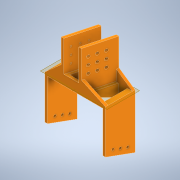
# Autodesk Inventor part: bracketForGarageV02
Saved by Autodesk Inventor 2022.1 (Build 261234020, 234B)
## iProperties
Created: 2021-10-20
Part Number: bracketForGarageV02
Material: PC/ABS Plastic
Document SubType Name: Modeling
Designer: robst
Density: 0.357273 g/cm^3
Appearance: Orange
Author: robst
Autodesk Inventor part; units mm, degrees
note: some values were not read from the file. Chosen so that the rebuilt part matches the saved one: direction of "HoleForLeftSideOf2x4"; direction of "HolesForRightSideOf2x4".
ref_plane "YZ Plane" through (0, 0, 0) normal (1, 0, 0) x (0, 1, 0)
ref_plane "XY Plane" through (0, 0, 0) normal (0, 0, 1) x (1, 0, 0)
sketch "Sketch8" plane through (0, 0, 0) normal (0, 1, 0) x (-1, 0, 0)
  line L0 (82, 40) -> (-82, 40)
  line L1 (-82, 40) -> (-82, -40)
  line L2 (-82, -40) -> (82, -40)
  line L3 (82, -40) -> (82, 40)
  line L4 (82, 40) -> (-82, -40) construction
  line L5 (-82, 40) -> (82, -40) construction
  point P0 (0, 0)
  dimension "d28" = 80
  dimension "d29" = 164
  constraints: 12 end point, 2 midpoint, 2 parallel, 1 horizontal, 1 perpendicular
  measures "d28" distance of L2.end L0.start
  measures "d29" distance between parallel lines of L1 L3
extrude "Extrusion8" add sketch "Sketch8" against normal blind 7
sketch "Sketch9" plane through (0, -7, 0) normal (0, -1, 0) x (1, 0, 0)
  line L0 (82, 40) -> (-82, 40) projected
  line L1 (-82, -40) -> (82, -40) projected
  line L2 (-82, 40) -> (-75, 40)
  line L3 (-75, 40) -> (-75, -40)
  line L4 (-75, -40) -> (-82, -40)
  line L5 (-82, -40) -> (-82, 40)
  line L6 (82, -40) -> (82, 40) projected
  line L7 (82, -40) -> (75, -40)
  line L8 (75, -40) -> (75, 40)
  line L9 (75, 40) -> (82, 40)
  line L10 (82, 40) -> (82, -40)
  point P0 (0, 0)
  point P1 (75, 40)
  point P2 (75, -40)
  point P3 (-82, -40)
  dimension "d32" = 7
  dimension "d33" = 7
  constraints: 16 end point, 4 parallel, 2 horizontal, 2 perpendicular, 2 point on line
  measures "d32" distance between parallel lines of L3 L5
  measures "d33" distance between parallel lines of L6 L8
extrude "armsForCameraCase" add sketch "Sketch9" along normal blind 140 contours L6 L1 L8 L0 | L3 L1 L5 L0
sketch "Sketch10" plane through (-75, -7, 40) normal (1, 0, 0) x (0, 0, -1)
  line L0 (0, 0) -> (80, 0)
  line L1 (80, 0) -> (80, -140)
  line L2 (80, -140) -> (0, -140)
  line L3 (0, 0) -> (0, -140)
  line L4 (0, 0) -> (80, -29.117619)
  line L5 (80, -29.117619) -> (80, 0)
  line L6 (80, 0) -> (0, 0)
  point P0 (40, 7)
  point P1 (40, -14.558809)
  dimension "d48" = 20
  constraints: 6 end point, 2 collinear, 1 midpoint, 1 point on line
  measures "d48" angle of L4 L0
extrude "Extrusion10" add sketch "Sketch10" along normal up to surface (150 mm away) contours L0 L1 L4
sketch "Sketch11" plane through (0, 0, 0) normal (0, 1, 0) x (1, 0, 0)
  line L0 (82, 40) -> (-82, 40)
  line L1 (-82, -40) -> (82, -40)
  line L2 (-82, 40) -> (-82, -40)
  line L3 (82, -40) -> (82, 40)
  line L4 (-31.037968, -40) -> (-9.602032, 40)
  line L5 (-9.602032, 40) -> (-16.848966, 40)
  line L6 (-75, 40) -> (75, 40)
  line L7 (-16.848966, 40) -> (-38.284901, -40)
  line L8 (-38.284901, -40) -> (-31.037968, -40)
  line L9 (-31.037968, -40) -> (-31.037968, 40) construction
  line L10 (0, -40) -> (0, 40) construction
  line L11 (9.602032, -40) -> (31.037968, 40)
  line L12 (31.037968, 40) -> (38.284901, 40)
  line L13 (38.284901, 40) -> (16.848966, -40)
  line L14 (16.848966, -40) -> (9.602032, -40)
  point P0 (0, 0)
  point P1 (0, -40)
  point P2 (0, -40)
  point P3 (-20.32, 0)
  point P4 (0, 0)
  point P5 (20.32, 0)
  point P6 (38.284901, 40)
  point P7 (31.037968, 40)
  point P8 (-16.848966, 40)
  dimension "d39" = -15
  dimension "d40" = 7
  dimension "d42" = 7
  dimension "d44" = 20.32
  dimension "d45" = 20.32
  constraints: 20 end point, 5 point on line, 4 midpoint, 3 parallel, 2 horizontal, 1 perpendicular, 8 other
  measures "d39" angle of L4 L9
  measures "d40" distance between parallel lines of L7 L4
  measures "d42" distance between parallel lines of L13 L11
  measures "d44" distance of point (-20.32, 0) point (0, 0)
  measures "d45" distance of point (20.32, 0) point (0, 0)
extrude "Extrusion11" add sketch "Sketch11" along normal blind 104.1375 contours L13 L1 L11 L0 | L4 L1 L7 L0
sketch "Sketch12" plane through (0, 0, 0) normal (0, 1, 0) x (1, 0, 0)
  line L0 (31.037968, 40) -> (-9.602032, 40)
  line L1 (31.037968, 40) -> (9.602032, -40)
  line L2 (-31.037968, -40) -> (9.602032, -40)
  line L3 (-31.037968, -40) -> (-9.602032, 40)
  line L4 (-9.602032, 40) -> (31.037968, 40)
  line L5 (31.037968, 40) -> (9.602032, -40)
  line L6 (9.602032, -40) -> (-31.037968, -40)
  line L7 (-9.602032, 40) -> (-31.037968, -40)
  line L8 (-31.037968, -40) -> (-9.602032, 40)
  point P0 (0, 0)
  constraints: 8 end point, 3 equal length
extrude "Extrusion12" add sketch "Sketch12" along normal blind 20
sketch "Sketch13" plane through (-82, 0, -40) normal (-1, 0, 0) x (0, 0, 1)
  line L0 (0, -36.117619) -> (80, -7)
  line L1 (80, 0) -> (80, -147)
  line L2 (80, -147) -> (0, -147)
  line L3 (0, 0) -> (0, -147)
  line L4 (80, -147) -> (0, -147) construction
  line L5 (40, -147) -> (40, -21.558809) construction
  line L6 (80, -7) -> (0, -36.117619) construction
  line L7 (0, -131.893618) -> (80, -102.776) construction
  line L8 (80, -7) -> (80, -147) construction
  point P0 (40, 0)
  point P1 (40, -117.334809)
  point P2 (20, -124.614214)
  point P3 (60, -110.055404)
  dimension "centerForTwoHoles" = 21.28356
  dimension "d51" = 90
  dimension "diagonalLine" = 85.13422
  dimension "d62" = 21.28356
  dimension "d63" = 21.28356
  constraints: 4 end point, 4 point on line, 3 midpoint, 1 parallel
  measures "d51" distance between parallel lines of L7 L0
  measures "diagonalLine" distance of L7.start L7.end
  measures "d62" distance of point (20, -124.614) L7.start
  measures "d63" distance of point (60, -110.055) L7.end
hole "Hole1" at (-82, -117.334809, 0) at (-82, -124.614214, -20) at (-82, -110.055404, 20) direction (1, 0, 0) diameter 6.7564 end through all clearance for "Hex Machine Screw" size "1/4" standard "Ansi Unified Screw Threads"
sketch "Sketch14" plane through (-82, 0, -40) normal (-1, 0, 0) x (0, 0, 1)
  line L0 (80, 0) -> (80, -147)
  line L1 (80, -147) -> (0, -147)
  line L2 (0, 0) -> (0, -147)
  line L3 (0, -36.117619) -> (80, -7)
  line L4 (0, -36.117619) -> (0, -147)
  line L5 (0, -147) -> (80, -117.882381)
  line L6 (0, -147) -> (80, -147)
  line L7 (0, -147) -> (80, -147)
  line L8 (80, -147) -> (80, -117.882381)
  point P0 (40, 0)
  constraints: 6 end point, 2 collinear, 1 parallel, 1 point on line
extrude "Extrusion13" cut sketch "Sketch14" against normal through all contours L0 L1 L5
sketch "Sketch15" plane through (-38.284901, 0, 40) normal (-0.9659258, 0, -0.258819) x (-0.258819, 0, 0.9659258)
  line L0 (-82.822094, 104.1375) -> (0, 104.1375)
  line L1 (0, 0) -> (0, 104.1375)
  line L2 (-82.822094, 0) -> (-82.822094, 104.1375)
  line L3 (-1.875644, 20) -> (-84.697739, 20)
  line L4 (-82.822094, 40) -> (0, 40) construction
  line L5 (-57.822094, 40) -> (-57.822094, 104.1375) construction
  point P0 (-48.545895, 0)
  point P1 (-82.822094, 52.06875)
  point P2 (-37.822094, 40)
  point P3 (-17.822094, 40)
  point P4 (-57.822094, 60)
  point P5 (-37.822094, 60)
  point P6 (-17.822094, 60)
  point P7 (-57.822094, 80)
  point P8 (-37.822094, 80)
  point P9 (-17.822094, 80)
  dimension "d64" = 25
  dimension "d74" = 20
  dimension "d77" = 20
  dimension "d90" = 20
  constraints: 4 end point, 4 point on line, 2 perpendicular, 1 coincident, 1 horizontal, 1 midpoint, 1 vertical, 8 other
  measures "d64" distance from line of point (-82.822, 52.069) L5
  measures "d74" distance of point (-57.822, 40) point (-37.822, 40)
  measures "d77" distance of point (-57.822, 40) point (-57.822, 60)
  measures "d90" distance between parallel lines of L4 L3
hole "HoleForLeftSideOf2x4" at (-23.319442, 40, -15.851854) at (-28.495823, 40, 3.466662) at (-33.672203, 40, 22.785179) at (-28.495823, 60, 3.466662) at (-23.319442, 60, -15.851854) at (-33.672203, 60, 22.785179) at (-33.672203, 80, 22.785179) at (-28.495823, 80, 3.466662) at (-23.319442, 80, -15.851854) direction (0.9659258, 0, 0.258819) diameter 4.496 depth 7 countersink diameter 8.433 countersink angle 82 clearance for "Flat Head Machine Screw (82)" size "#8" standard "Ansi Unified Screw Threads"
sketch "Sketch16" plane through (38.284901, 0, -40) normal (0.9659258, 0, 0.258819) x (0.258819, 0, -0.9659258)
  line L0 (-82.822094, 104.1375) -> (0, 104.1375)
  line L1 (0, 0) -> (0, 104.1375)
  line L2 (-82.822094, 0) -> (-82.822094, 104.1375)
  line L3 (-82.822094, 0) -> (-65.959766, 0)
  line L4 (-1.875644, 20) -> (-84.697739, 20)
  line L5 (-82.822094, 40) -> (0, 40) construction
  line L6 (-67.822094, 40) -> (-67.822094, 104.1375) construction
  point P0 (-48.545895, 0)
  point P1 (-47.822094, 40)
  point P2 (-27.822094, 40)
  point P3 (-67.822094, 60)
  point P4 (-47.822094, 60)
  point P5 (-27.822094, 60)
  point P6 (-67.822094, 80)
  point P7 (-47.822094, 80)
  point P8 (-27.822094, 80)
  dimension "d80" = 20
  dimension "d81" = 15
  dimension "d84" = 20
  dimension "d87" = 20
  constraints: 4 end point, 4 point on line, 2 perpendicular, 1 coincident, 1 horizontal, 1 vertical, 8 other
  measures "d80" distance between parallel lines of L5 L4
  measures "d81" distance between parallel lines of L6 L2
  measures "d84" distance of point (-67.822, 40) point (-47.822, 40)
  measures "d87" distance of point (-67.822, 40) point (-67.822, 60)
hole "HolesForRightSideOf2x4" at (25.907632, 40, 6.192596) at (31.084013, 40, -13.12592) at (20.731251, 60, 25.511113) at (25.907632, 60, 6.192596) at (31.084013, 60, -13.12592) at (20.731251, 80, 25.511113) at (25.907632, 80, 6.192596) at (31.084013, 80, -13.12592) at (20.731251, 40, 25.511113) direction (-0.9659258, 0, -0.258819) diameter 4.496 depth 7 countersink diameter 8.433 countersink angle 82 clearance for "Flat Head Machine Screw (82)" size "#8" standard "Ansi Unified Screw Threads"
sketch "Sketch17" plane through (0, 20, 0) normal (0, 1, 0) x (1, 0, 0)
  line L0 (31.037968, 40) -> (9.602032, -40)
  line L1 (-31.037968, -40) -> (9.602032, -40)
  line L2 (-31.037968, -40) -> (-9.602032, 40)
  line L3 (31.037968, 40) -> (-9.602032, 40)
  line L4 (21.91539, 33) -> (4.230743, -33)
  line L5 (4.230743, -33) -> (-21.91539, -33)
  line L6 (-21.91539, -33) -> (-4.230743, 33)
  line L7 (-4.230743, 33) -> (21.91539, 33)
  point P0 (0, 0)
  point P1 (10.717968, 40)
  point P2 (-8.842323, -33)
  dimension "d98" = 7
  dimension "d99" = 7
  dimension "d101" = 7
  dimension "d102" = 7
  constraints: 8 end point, 4 parallel, 2 midpoint, 1 horizontal
  measures "d98" distance between parallel lines of L4 L0
  measures "d99" distance between parallel lines of L6 L2
  measures "d101" distance from line of point (10.718, 40) L7
  measures "d102" distance from line of point (-8.842, -33) L1
extrude "Extrusion14" cut sketch "Sketch17" against normal through all contours L4 L5 L6 L7
sketch "Sketch18" plane through (0, 0, 0) normal (0, 1, 0) x (1, 0, 0)
  line L0 (16.848966, -40) -> (82, -40)
  line L1 (16.848966, -40) -> (38.284901, 40)
  line L2 (82, 40) -> (38.284901, 40)
  line L3 (82, -40) -> (82, 40)
  line L4 (68, -33) -> (68, 33)
  line L5 (68, 33) -> (43.65619, 33)
  line L6 (43.65619, 33) -> (25.971543, -33)
  line L7 (25.971543, -33) -> (68, -33)
  line L8 (38.284901, 40) -> (16.848966, -40)
  line L9 (16.848966, -40) -> (82, -40)
  line L10 (82, -40) -> (82, 40)
  line L11 (82, 40) -> (38.284901, 40)
  point P0 (0, 0)
  dimension "d105" = 7
  dimension "d107" = 7
  dimension "d108" = 14
  dimension "d109" = 7
  constraints: 8 end point, 4 parallel, 1 perpendicular
  measures "d105" distance between parallel lines of L7 L0
  measures "d107" distance between parallel lines of L1 L6
  measures "d108" distance between parallel lines of L3 L4
  measures "d109" distance between parallel lines of L5 L2
extrude "Extrusion15" cut sketch "Sketch18" against normal through all contours L7 L6 L5 L4
sketch "Sketch19" plane through (0, 0, 0) normal (0, 1, 0) x (1, 0, 0)
  line L0 (-16.848966, 40) -> (-38.284901, -40)
  line L1 (-82, -40) -> (-38.284901, -40)
  line L2 (-82, 40) -> (-82, -40)
  line L3 (-16.848966, 40) -> (-82, 40)
  line L4 (-25.971543, 33) -> (-43.65619, -33)
  line L5 (-43.65619, -33) -> (-68, -33)
  line L6 (-68, -33) -> (-68, 33)
  line L7 (-68, 33) -> (-25.971543, 33)
  point P0 (0, 0)
  point P1 (-60.14245, -40)
  dimension "d112" = 7
  dimension "d113" = 14
  dimension "d114" = 7
  dimension "d115" = 7
  constraints: 8 end point, 4 parallel, 1 horizontal, 1 midpoint
  measures "d112" distance between parallel lines of L0 L4
  measures "d113" distance between parallel lines of L6 L2
  measures "d114" distance from line of point (-60.142, -40) L5
  measures "d115" distance between parallel lines of L3 L7
extrude "Extrusion16" cut sketch "Sketch19" against normal through all contours L4 L5 L6 L7
sketch "Sketch27" plane through (-75, -7, 40) normal (0, 0, 1) x (1, 0, 0)
  line L0 (91.848966, 7) -> (157, 7)
  line L1 (91.848966, 7) -> (91.848966, 111.1375)
  line L2 (157, 7) -> (157, -110.882381)
  line L3 (91.848966, 37) -> (157, 7)
  line L4 (157, 7) -> (91.848966, 7)
  line L5 (91.848966, 7) -> (91.848966, 37)
  point P0 (75, 7)
  dimension "d152" = 30
  constraints: 6 end point, 2 collinear, 1 point on line
  measures "d152" distance of L0.start L3.start
sketch "Sketch28" plane through (68, 0, 33) normal (0, 0, -1) x (-1, 0, 0)
  line L0 (-14, 0) -> (49.939383, 0)
  line L1 (51.151034, 0) -> (51.151034, 104.1375)
  line L2 (49.939383, 0) -> (49.939383, 30)
  line L3 (49.939383, 30) -> (-14, 0)
  point P0 (68, 0)
  dimension "d153" = 30
  constraints: 6 end point, 1 parallel, 1 perpendicular
  measures "d153" distance of L0.end L2.end
loft "Loft5" add profiles "Sketch27", "Sketch28"
sketch "Sketch29" plane through (75, -36.117619, -40) normal (0, 0, -1) x (-1, 0, 0)
  line L0 (-7, 36.117619) -> (36.715099, 36.117619)
  line L1 (36.715099, 36.117619) -> (36.715099, 140.255119)
  line L2 (-7, 36.117619) -> (-7, -81.764763)
  line L3 (-7, 36.117619) -> (36.715099, 36.117619)
  line L4 (36.715099, 36.117619) -> (36.715099, 66.117619)
  line L5 (36.715099, 66.117619) -> (-7, 36.117619)
  point P0 (75, 36.117619)
  dimension "d158" = 30
  constraints: 6 end point, 1 collinear, 1 point on line
  measures "d158" distance of L4.end L0.end
sketch "Sketch30" plane through (43.65619, 0, -33) normal (0, 0, 1) x (1, 0, 0)
  line L0 (-5.371289, 0) -> (-5.371289, 104.1375)
  line L1 (38.34381, 0) -> (-5.371289, 0)
  line L2 (-5.371289, 0) -> (-5.371289, 104.1375)
  line L3 (-5.371289, 0) -> (38.34381, 0)
  line L4 (38.34381, 0) -> (-5.371289, 30)
  line L5 (-5.371289, 30) -> (-5.371289, 0)
  point P0 (-43.65619, 0)
  dimension "d159" = 30
  constraints: 6 end point, 1 collinear, 1 perpendicular, 1 point on line
  measures "d159" distance of L4.end L0.start
loft "Loft6" add profiles "Sketch29", "Sketch30"
sketch "Sketch31" plane through (-75, -7, 40) normal (0, 0, 1) x (1, 0, 0)
  line L0 (-7, 7) -> (36.715099, 7)
  line L1 (36.715099, 7) -> (36.715099, 111.1375)
  line L2 (58.151034, 7) -> (-7, 7)
  line L3 (-7, 7) -> (36.715099, 7)
  line L4 (36.715099, 7) -> (36.715099, 46)
  line L5 (36.715099, 46) -> (-7, 7)
  point P0 (75, 7)
  dimension "d164" = 39
  constraints: 6 end point, 1 horizontal, 1 point on line
  measures "d164" distance of L4.end L0.end
sketch "Sketch32" plane through (-43.65619, 0, 33) normal (0, 0, -1) x (-1, 0, 0)
  line L0 (38.34381, 0) -> (-5.371289, 0)
  line L1 (38.34381, 0) -> (-7.943181, 0)
  line L2 (-7.943181, 0) -> (-7.943181, 30)
  line L3 (-7.943181, 30) -> (38.34381, 0)
  point P0 (-43.65619, 0)
  dimension "d165" = 30
  constraints: 6 end point, 1 horizontal, 1 perpendicular
  measures "d165" distance of L1.end L2.end
sketch "Sketch31 outline for Loft7" plane through (-75, -7, 40) normal (0, 0, 1) x (1, 0, 0)
  line L0 (36.715099, 46) -> (-7, 7)
  line L1 (36.715099, 7) -> (36.715099, 46)
  line L2 (-7, 7) -> (36.715099, 7)
sketch "Sketch32 outline for Loft7" plane through (-43.65619, 0, 33) normal (0, 0, -1) x (-1, 0, 0)
  line L0 (38.34381, 0) -> (-7.943181, 0)
  line L1 (-7.943181, 0) -> (-7.943181, 30)
  line L2 (-7.943181, 30) -> (38.34381, 0)
loft "Loft7" add profiles "Sketch31 outline for Loft7", "Sketch32 outline for Loft7"
sketch "Sketch33" plane through (75, -36.117619, -40) normal (0, 0, -1) x (-1, 0, 0)
  line L0 (91.848966, 36.117619) -> (157, 36.117619)
  line L1 (91.848966, 36.117619) -> (91.848966, 140.255119)
  line L2 (111.409257, 36.117619) -> (91.848966, 36.117619)
  line L3 (91.848966, 36.117619) -> (157, 36.117619)
  line L4 (157, 36.117619) -> (91.848966, 66.117619)
  line L5 (91.848966, 66.117619) -> (91.848966, 36.117619)
  point P0 (75, 36.117619)
  dimension "d171" = 30
  constraints: 6 end point, 2 collinear, 1 point on line
  measures "d171" distance of L4.end L0.start
sketch "Sketch34" plane through (-68, 0, -33) normal (0, 0, 1) x (1, 0, 0)
  line L0 (51.151034, 0) -> (-14, 0)
  line L1 (51.151034, 0) -> (51.151034, 104.1375)
  line L2 (-14, 0) -> (50.026246, 0)
  line L3 (31.590743, 0) -> (51.151034, 0)
  line L4 (50.026246, 0) -> (50.026246, 30)
  line L5 (50.026246, 30) -> (-14, 0)
  point P0 (68, 0)
  dimension "d170" = 30
  constraints: 6 end point, 1 point on line, 1 vertical
  measures "d170" distance of L2.end L4.end
loft "Loft8" add profiles "Sketch33", "Sketch34"
equation "\"d28\" = widthOfBracket"
equation "\"d30\" = wallThickness"
equation "\"d32\" = wallThickness"
equation "\"d33\" = wallThickness"
equation "\"d34\" = bracketLength"
equation "\"d48\" = elevation"
equation "\"d39\" = azimuth"
equation "\"d40\" = wallThickness"
equation "\"d42\" = wallThickness"
equation "\"d44\" = 0.5 * twoByFourWidth"
equation "\"d45\" = 0.5 * twoByFourWidth"
equation "\"d46\" = twoByFourDepth + baseBelowTwoByFour"
equation "\"d49\" = baseBelowTwoByFour"
equation "\"centerForTwoHoles\" = 0.25 * diagonalLine"
equation "\"d62\" = centerForTwoHoles"
equation "\"d63\" = centerForTwoHoles"
equation "\"d98\" = wallThickness"
equation "\"d99\" = wallThickness"
equation "\"d101\" = wallThickness"
equation "\"d102\" = wallThickness"
equation "\"d105\" = wallThickness"
equation "\"d107\" = wallThickness"
equation "\"d108\" = 2 * wallThickness"
equation "\"d109\" = wallThickness"
equation "\"d112\" = wallThickness"
equation "\"d113\" = 2 * wallThickness"
equation "\"d114\" = wallThickness"
equation "\"d115\" = wallThickness"
equation "\"wallThickness\" = 7"
equation "\"widthOfBracket\" = 80"
equation "\"twoByFourWidth\" = 40.64"
equation "\"twoByFourDepth\" = 84.1375"
equation "\"azimuth\" = -15deg"
equation "\"elevation\" = 20deg"
equation "\"baseBelowTwoByFour\" = 20"
equation "\"bracketLength\" = 140"
body "Solid2"
